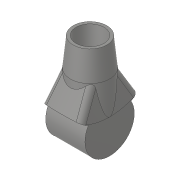
# Autodesk Inventor part: GRIP_BASE_V2
Saved by Autodesk Inventor 2019.4 (Build 234330000, 330)
## iProperties
Created: 2019-12-04
Part Number: GRIP_BASE_V2
Material: 一般
Document SubType Name: Modeling
Designer: y6tada
Density: 1 g/cm^3
Appearance: 滑らか - 標準の灰色
Author: y6tada
Autodesk Inventor part; units mm, degrees
ref_plane "YZ Plane" through (0, 0, 0) normal (1, 0, 0) x (0, 1, 0)
ref_plane "XZ Plane" through (0, 0, 0) normal (0, 1, 0) x (-1, 0, 0)
ref_plane "XY Plane" through (0, 0, 0) normal (0, 0, 1) x (1, 0, 0)
sketch "スケッチ4" plane through (0, 0, 0) normal (1, 0, 0) x (0, 1, 0)
  line L0 (0, 0) -> (45.0295, 0) construction
  arc A0 (6.1, 10.5655) -> (6.1, -10.5655) centre (0, 0) ccw
  line L1 (6.1, 10.5655) -> (24.4, 0)
  line L2 (6.1, -10.5655) -> (24.4, 0)
  dimension "d15" = 12.2
  dimension "d16" = 60
  constraints: 6 end point, 2 point on circle, 2 tangent, 1 centre point, 1 coincident, 1 horizontal, 1 point on line
  measures "d15" radius of A0
  measures "d16" angle of L2 L1
extrude "押し出し2" add sketch "スケッチ4" along normal mid plane 14
sketch "スケッチ5" plane through (0, 0, 0) normal (0, 0, 1) x (1, 0, 0)
  arc A0 (-7.1, -11.5) -> (7.1, -11.5) centre (0, 24.1571) ccw
  line L0 (-7, -12.2) -> (7, -12.2) construction
  line L1 (0, 0) -> (0, 26.1407) construction
  line L2 (-7.1, -11.5) -> (-7.1, -15.2)
  line L3 (-7.1, -15.2) -> (7.1, -15.2)
  line L4 (7.1, -15.2) -> (7.1, -11.5)
  dimension "d19" = 11.5
  dimension "d20" = 3
  dimension "d23" = 14.2
  dimension "d40" = 12.2
  constraints: 8 end point, 3 vertical, 2 point on circle, 1 centre point, 1 horizontal, 1 point on line, 1 tangent, 1 other
  measures "d19" vertical distance of L4.end L1.start
  measures "d20" distance between parallel lines of L3 L0
  measures "d23" distance of L2.end L3.end
  measures "d40" distance from line of L1.start L0
sketch "スケッチ6" plane through (7, 0, 0) normal (1, 0, 0) x (0, 0, -1)
  arc A0 (-10.5655, 6.1) -> (10.5655, 6.1) centre (0, 0) ccw projected
  line L0 (10.5655, 6.1) -> (0, 24.4) projected
  line L1 (0, 24.4) -> (-10.5655, 6.1) projected
sketch "スケッチ8" plane through (0, 6.1, 10.5655) normal (0, 0.5, 0.8660254) x (1, 0, 0)
  line L0 (4.5, 21.131) -> (7, 21.131)
  line L1 (7, 21.131) -> (7, 0)
  line L2 (7, 0) -> (4.5, 21.131)
  line L3 (0, 0) -> (7, 0) construction
  line L4 (-7, 21.131) -> (7, 21.131) construction
  line L5 (0, 0) -> (0, 28.6772) construction
  line L6 (-4.5, 21.131) -> (-7, 21.131)
  line L7 (-7, 21.131) -> (-7, 0)
  line L8 (-7, 0) -> (-4.5, 21.131)
  dimension "d27" = 2.5
  constraints: 16 end point, 2 horizontal, 2 symmetric about line, 2 vertical
  measures "d27" distance of L0.start L0.end
revolve "回転3" cut sketch "スケッチ8" angle 360 about axis through (-7, 24.4, 0) along (1, 0, 0)
sketch3d "3D スケッチ1"
  line L0 (7, 6.1, 10.5655) -> (7, 24.4, 0)
  line L1 (7, 24.4, 0) -> (7, 6.1, -10.5655)
  arc A0 (7, 6.1, 10.5655) -> (7, -6.1, 10.5655) centre (7, 0, 0) ccw
  arc A1 (7, -6.1, 10.5655) -> (7, -12.2, 0) centre (7, 0, 0) ccw
  arc A2 (7, -12.2, 0) -> (7, -6.1, -10.5655) centre (7, 0, 0) ccw
  arc A3 (7, -6.1, -10.5655) -> (7, 6.1, -10.5655) centre (7, 0, 0) ccw
sweep "スイープ1" cut profiles "スケッチ5" path "3D スケッチ1"
sketch "スケッチ7" plane through (0, 0, 0) normal (0, 1, 0) x (-1, 0, 0)
  circle A0 centre (0, 0) radius 7
  dimension "d24" = 14
  constraints: 1 centre point, 1 coincident
  measures "d24" diameter of A0
extrude "押し出し3" add sketch "スケッチ7" along normal blind 25
sketch "スケッチ9" plane through (0, 0, 0) normal (0, 0, 1) x (1, 0, 0)
  line L0 (-7.5, -8.8) -> (7.5, -8.8)
  line L1 (7.5, -8.8) -> (7.5, -13.8)
  line L2 (7.5, -13.8) -> (-7.5, -13.8)
  line L3 (-7.5, -13.8) -> (-7.5, -8.8)
  line L4 (0, 0) -> (0, -19.5506) construction
  line L5 (0, 0) -> (28.6697, 0) construction
  dimension "d29" = 15
  dimension "d30" = 5
  dimension "d31" = 8.8
  constraints: 12 end point, 2 horizontal, 2 parallel, 1 perpendicular, 1 vertical, 1 other
  measures "d29" distance of L1.end L2.end
  measures "d30" distance of L0.end L1.end
  measures "d31" distance from line of L4.start L0
revolve "回転4" cut sketch "スケッチ9" angle 240 mid plane about axis through (0, 0, 0) along (1, 0, 0)
sketch "スケッチ10" plane through (0, 0, 0) normal (0, 1, 0) x (1, 0, 0)
  circle A0 centre (0, 0) radius 5
  dimension "d33" = 10
  constraints: 1 centre point, 1 coincident
  measures "d33" diameter of A0
extrude "押し出し4" cut sketch "スケッチ10" along normal through all
fillet "フィレット1" radius 2 4 edges at (-6.2937, 11.0044, 7.1002) (6.2937, 11.0044, 7.1002) (6.2937, 11.0044, -7.1002) (-6.2937, 11.0044, -7.1002)
chamfer "面取り1" distance 1 distance2 10 1 edges at (7, 25, 0) measured on face at (6.5, 25, 0)
